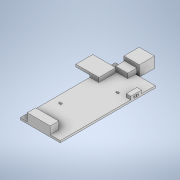
# Autodesk Inventor part: esp32_t8
Saved by Autodesk Inventor 2020 (Build 240168000, 168)
## iProperties
Created: 2020-03-15
Part Number: esp32_t8
Material: Generic
Document SubType Name: Modeling
Designer: erwin
Density: 1 g/cm^3
Appearance: Default
Author: erwin
Autodesk Inventor part; units mm, degrees
ref_plane "YZ Plane" through (0, 0, 0) normal (1, 0, 0) x (0, 1, 0)
ref_plane "XZ Plane" through (0, 0, 0) normal (0, 1, 0) x (-1, 0, 0)
ref_plane "XY Plane" through (0, 0, 0) normal (0, 0, 1) x (1, 0, 0)
sketch "Sketch1" plane through (0, 0, 0) normal (0, 1, 0) x (-1, 0, 0)
  line L0 (-13, -31) -> (13, -31)
  line L1 (13, -31) -> (13, 31)
  line L2 (13, 31) -> (-13, 31)
  line L3 (-13, 31) -> (-13, -31)
  line L4 (-13, -31) -> (13, 31) construction
  line L5 (13, -31) -> (-13, 31) construction
  point P0 (0, 0)
  dimension "d0" = 26
  dimension "d1" = 62
  constraints: 12 end point, 2 midpoint, 2 parallel, 1 horizontal, 1 perpendicular
  measures "d0" distance of L2.end L1.end
  measures "d1" distance of L1.end L0.end
extrude "Extrusion1" add sketch "Sketch1" along normal blind 1.3
sketch "Sketch2" plane through (0, 1.3, 0) normal (0, 1, 0) x (1, 0, 0)
  line L0 (-8, 26) -> (0, 26)
  line L1 (0, 26) -> (0, 32)
  line L2 (0, 32) -> (-8, 32)
  line L3 (-8, 32) -> (-8, 26)
  line L4 (13, 31) -> (-13, 31) projected
  line L5 (-13, 31) -> (-13, -31) projected
  point P0 (0, 0)
  dimension "d4" = 8
  dimension "d5" = 6
  dimension "d6" = 1
  dimension "d7" = 5
  constraints: 8 end point, 2 parallel, 1 horizontal, 1 perpendicular
  measures "d4" distance of L2.end L1.end
  measures "d5" distance of L1.end L0.end
  measures "d6" distance between parallel lines of L4 L2
  measures "d7" distance between parallel lines of L5 L3
extrude "Extrusion2" add sketch "Sketch2" along normal blind 3
sketch "Sketch3" plane through (-13, 0, -31) normal (-1, 0, 0) x (0, 0, 1)
  line L0 (16.6, 2.6) -> (5.6, 2.6)
  line L1 (5.6, 2.6) -> (5.6, 4.1)
  line L2 (5.6, 4.1) -> (16.6, 4.1)
  line L3 (16.6, 4.1) -> (16.6, 2.6)
  line L4 (0, 0) -> (62, 0) projected
  line L5 (0, 0) -> (0, 1.3) projected
  point P0 (31, 0)
  dimension "d10" = 11
  dimension "d11" = 1.5
  dimension "d12" = 2.6
  dimension "d13" = 5.6
  constraints: 8 end point, 2 parallel, 1 horizontal, 1 perpendicular
  measures "d10" distance of L1.end L2.end
  measures "d11" distance of L0.end L1.end
  measures "d12" distance between parallel lines of L4 L0
  measures "d13" distance between parallel lines of L5 L1
extrude "Extrusion3" add sketch "Sketch3" along normal blind 9.2 and the other way blind 5.8
sketch "Sketch4" plane through (0, 1.3, 0) normal (0, 1, 0) x (1, 0, 0)
  line L0 (-13, 31) -> (-13, -31) projected
  line L1 (-7.2, 25.4) -> (-22.2, 25.4) projected
  line L2 (-7.2, 14.4) -> (-22.2, 14.4) projected
  line L3 (-7.2, 25.4) -> (-13, 25.4)
  line L4 (-13, 25.4) -> (-13, 14.4)
  line L5 (-13, 14.4) -> (-7.2, 14.4)
  line L6 (-7.2, 14.4) -> (-7.2, 25.4)
  point P0 (0, 0)
  point P1 (-13, 25.4)
  constraints: 8 end point, 2 parallel, 2 point on line, 1 horizontal, 1 perpendicular
extrude "Extrusion4" add sketch "Sketch4" along normal up to surface (2.8 mm away)
sketch "Sketch5" plane through (13, 0, 31) normal (1, 0, 0) x (0, 0, -1)
  line L0 (46, 3.3) -> (53, 3.3)
  line L1 (53, 3.3) -> (53, 1.3)
  line L2 (53, 1.3) -> (46, 1.3)
  line L3 (46, 1.3) -> (46, 3.3)
  line L4 (0, 1.3) -> (62, 1.3) projected
  line L5 (62, 0) -> (62, 1.3) projected
  point P0 (31, 0)
  dimension "d20" = 16
  dimension "d21" = 7
  dimension "d22" = 2
  constraints: 8 end point, 2 parallel, 1 collinear, 1 horizontal, 1 perpendicular
  measures "d20" distance between parallel lines of L5 L3
  measures "d21" distance of L0.start L0.end
  measures "d22" distance of L0.end L1.end
extrude "Extrusion5" add sketch "Sketch5" against normal blind 3
sketch "Sketch6" plane through (13, 0, 31) normal (1, 0, 0) x (0, 0, -1)
  line L0 (48, 2.5) -> (49.2, 2.5)
  line L1 (49.2, 2.5) -> (49.2, 1.5)
  line L2 (49.2, 1.5) -> (48, 1.5)
  line L3 (48, 1.5) -> (48, 2.5)
  line L4 (62, 0) -> (62, 1.3) projected
  line L5 (0, 0) -> (62, 0) projected
  point P0 (31, 0)
  dimension "d25" = 1.2
  dimension "d26" = 1
  dimension "d27" = 14
  dimension "d28" = 2.5
  constraints: 8 end point, 2 parallel, 1 horizontal, 1 perpendicular
  measures "d25" distance of L1.end L2.end
  measures "d26" distance of L0.end L1.end
  measures "d27" distance between parallel lines of L4 L3
  measures "d28" distance between parallel lines of L5 L0
extrude "Extrusion6" add sketch "Sketch6" along normal blind 0.5
pattern_linear "Rectangular Pattern1" count 2 spacing 1.5 along (0, 0, -1) of "Extrusion6"
sketch "Sketch7" plane through (0, 1.3, -32) normal (0, 0, -1) x (-1, 0, 0)
  line L0 (0, 0) -> (8, 0) projected
  line L1 (8, 0) -> (8, 3) projected
  line L2 (0, 3) -> (8, 3) projected
  line L3 (0, 0) -> (0, 3) projected
  line L4 (7.5, 2.5) -> (7.5, 0.5)
  line L5 (7.5, 0.5) -> (0.5, 0.5)
  line L6 (0.5, 0.5) -> (0.5, 2.5)
  line L7 (0.5, 2.5) -> (7.5, 2.5)
  point P0 (0, -1.3)
  dimension "d34" = 0.5
  constraints: 8 end point, 3 other
  measures "d34" distance between parallel lines of L2 L7
extrude "Extrusion7" add sketch "Sketch7" along normal blind 0.5 contours L4 L5 L6 L7
sketch "Sketch8" plane through (0, 1.3, -32.5) normal (0, 0, -1) x (-1, 0, 0)
  line L0 (7.5, 2.5) -> (0.5, 2.5) projected
  line L1 (0.5, 2.5) -> (0.5, 0.5) projected
  line L2 (0.5, 0.5) -> (7.5, 0.5) projected
  line L3 (7.5, 0.5) -> (7.5, 2.5) projected
  line L4 (9, 5) -> (-1, 5)
  line L5 (-1, 5) -> (-1, -2)
  line L6 (-1, -2) -> (9, -2)
  line L7 (9, -2) -> (9, 5)
  line L8 (9, 5) -> (-1, -2) construction
  line L9 (-1, 5) -> (9, -2) construction
  point P0 (0, -1.3)
  point P1 (4, 1.5)
  dimension "d37" = 10
  dimension "d38" = 7
  constraints: 12 end point, 2 midpoint, 2 parallel, 1 horizontal, 1 perpendicular
  measures "d37" distance of L6.end L5.end
  measures "d38" distance of L5.end L4.end
extrude "Extrusion8" add sketch "Sketch8" along normal blind 10 contours L3 L2 L1 L0 | L7 L6 L5 L4
sketch "Sketch9" plane through (0, 1.3, 0) normal (0, 1, 0) x (1, 0, 0)
  line L0 (-13, -31) -> (13, -31) projected
  line L1 (-8.5, -31) -> (6.5, -31)
  line L2 (6.5, -31) -> (6.5, -25.5)
  line L3 (6.5, -25.5) -> (-8.5, -25.5)
  line L4 (-8.5, -25.5) -> (-8.5, -31)
  line L5 (-13, 14.4) -> (-13, -31) projected
  point P0 (0, 0)
  dimension "d41" = 15
  dimension "d42" = 5.5
  dimension "d43" = 4.5
  constraints: 8 end point, 2 parallel, 1 horizontal, 1 perpendicular, 1 point on line
  measures "d41" distance of L3.end L2.end
  measures "d42" distance of L2.end L1.end
  measures "d43" distance between parallel lines of L4 L5
extrude "Extrusion9" add sketch "Sketch9" along normal blind 5
sketch "Sketch10" plane through (0, 1.3, 0) normal (0, 1, 0) x (1, 0, 0)
  line L0 (-8.5, -10.5) -> (-7.1, -10.5)
  line L1 (-7.1, -10.5) -> (-7.1, -9.7)
  line L2 (-7.1, -9.7) -> (-8.5, -9.7)
  line L3 (-8.5, -9.7) -> (-8.5, -10.5)
  line L4 (-13, 14.4) -> (-13, -31) projected
  line L5 (-13, -31) -> (-8.5, -31) projected
  line L6 (5.5, 15) -> (4.1, 15)
  line L7 (4.1, 15) -> (4.1, 14.2)
  line L8 (4.1, 14.2) -> (5.5, 14.2)
  line L9 (5.5, 14.2) -> (5.5, 15)
  line L10 (13, -31) -> (13, 15) projected
  line L11 (13, 31) -> (0, 31) projected
  point P0 (0, 0)
  dimension "d46" = 4.5
  dimension "d47" = 20.5
  dimension "d48" = 0.8
  dimension "d49" = 1.4
  dimension "d50" = 7.5
  dimension "d51" = 16
  dimension "d52" = 0.8
  dimension "d53" = 1.4
  constraints: 16 end point, 4 parallel, 2 horizontal, 2 perpendicular
  measures "d46" distance between parallel lines of L4 L3
  measures "d47" distance between parallel lines of L5 L0
  measures "d48" distance of L2.end L0.start
  measures "d49" distance of L1.end L2.end
  measures "d50" distance between parallel lines of L10 L9
  measures "d51" distance between parallel lines of L11 L6
  measures "d52" distance of L6.end L7.end
  measures "d53" distance of L7.end L8.end
extrude "Extrusion10" add sketch "Sketch10" along normal blind 0.5
equation "\"d52\" = d48"
equation "\"d53\" = d49"
body "Solid1"
